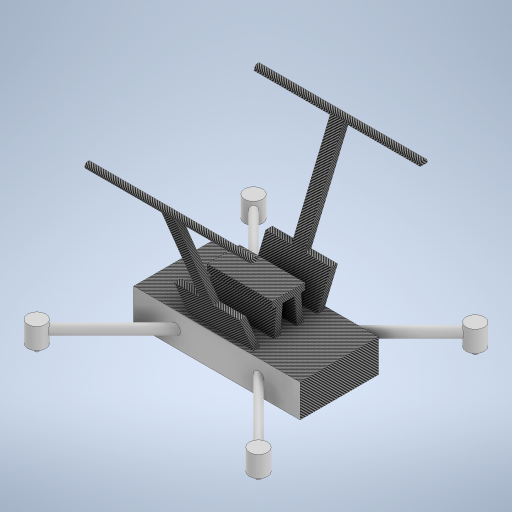
# Autodesk Inventor part: Drone_Model
Saved by Autodesk Inventor 2023 (Build 270158000, 158)
## iProperties
Created: 2022-11-14
Part Number: Drone_Model
Material: Generic
Document SubType Name: Modeling
Designer: cheng
Density: 1 g/cm^3
Appearance: Default
Mass: 1853.08 g
Surface Area: 1828.35 cm^2
Volume: 1853.08 cm^3
Author: cheng
Autodesk Inventor part; units mm, degrees
ref_plane "YZ Plane" through (0, 0, 0) normal (1, 0, 0) x (0, 1, 0)
ref_plane "XZ Plane" through (0, 0, 0) normal (0, 1, 0) x (-1, 0, 0)
sketch "Sketch4" plane through (0, 0, 0) normal (0, 1, 0) x (-1, 0, 0)
  line L0 (-102.6818, 131.0909) -> (-102.6818, 58.0909) construction
  line L1 (24.8182, 125) -> (-230.1818, 125)
  line L2 (-230.1818, 125) -> (-230.1818, 135)
  line L3 (-230.1818, 135) -> (24.8182, 135)
  line L4 (24.8182, 135) -> (24.8182, 125)
  line L5 (24.8182, 125) -> (-230.1818, 135) construction
  line L6 (-230.1818, 125) -> (24.8182, 135) construction
  line L7 (0, 0) -> (36.133, 0) construction
  line L8 (24.8182, -125) -> (-230.1818, -125)
  line L9 (-230.1818, -125) -> (-230.1818, -135)
  line L10 (-230.1818, -135) -> (24.8182, -135)
  line L11 (24.8182, -135) -> (24.8182, -125)
  line L12 (24.8182, -125) -> (-230.1818, -135) construction
  line L13 (-230.1818, -125) -> (24.8182, -135) construction
  point P0 (-102.6818, 130)
  dimension "d4" = 10
  dimension "d6" = 250
  dimension "d7" = 255
  constraints: 28 end point, 4 symmetric about line, 2 horizontal, 2 midpoint, 2 parallel, 1 perpendicular, 1 point on line, 1 vertical
  measures "d4" distance of L3.end L1.start
  measures "d6" distance between parallel lines of L8 L1
  measures "d7" distance of L2.end L3.end
extrude "Extrusion2" add sketch "Sketch4" along normal blind 10
sketch "Sketch9" plane through (230.1818, 0, -125) normal (1, 0, 0) x (0, 0, -1)
  line L0 (-125, 0) -> (-125, -106.9842) construction
  line L1 (10, 0) -> (10, 10) construction
  line L2 (0, 10) -> (10, 10) construction
  line L3 (10, 0) -> (0, 10) construction
  line L4 (0, 10) -> (10, 10) construction
  line L5 (10, 10) -> (0, 0) construction
  circle A0 centre (5, 5) radius 5
  line L6 (-260, 0) -> (-260, 10) construction
  line L7 (-250, 10) -> (-260, 10) construction
  line L8 (-260, 0) -> (-250, 10) construction
  line L9 (-250, 10) -> (-260, 10) construction
  line L10 (-260, 10) -> (-250, 0) construction
  circle A1 centre (-255, 5) radius 5
  constraints: 18 end point, 5 symmetric about line, 2 centre point, 1 collinear, 1 midpoint, 1 tangent, 1 vertical, 1 other
extrude "Extrusion3" cut sketch "Sketch9" against normal through all keep common part
sketch "Sketch10" plane through (230.1818, 5, -130) normal (1, 0, 0) x (0, 0, -1)
  circle A0 centre (0, 0) radius 5 construction
  line L0 (0, 5) -> (-260, 5)
  line L1 (-130, -5) -> (-130, 5) construction
  line L2 (-155, -155.4301) -> (-105, -155.4301)
  line L3 (-105, -155.4301) -> (-105, -145)
  line L4 (-105, -145) -> (-155, -145)
  line L5 (-155, -145) -> (-155, -155.4301)
  line L6 (-155, -155.4301) -> (-105, -145) construction
  line L7 (-105, -155.4301) -> (-155, -145) construction
  line L8 (-130, -150.215) -> (-130, -124.8826) construction
  dimension "d13" = 150
  dimension "d34" = 50
  constraints: 18 end point, 3 horizontal, 3 midpoint, 2 parallel, 1 collinear, 1 perpendicular, 1 vertical, 1 vertical alignment, 1 other
  measures "d13" distance between parallel lines of L4 L0
  measures "d34" distance of L2.start L2.end
extrude "Extrusion4" add sketch "Sketch10" against normal blind 255
sketch "Sketch11" plane through (230.1818, 5, -130) normal (1, 0, 0) x (0, 0, -1)
  circle A0 centre (0, 0) radius 5 projected
  line L0 (-155, -145) -> (-105, -145) projected
  line L1 (-130, 0) -> (-130, -145) construction
  line L2 (-130, -145) -> (-286.0792, -145) construction
  line L3 (-130, -145) -> (0, -145) construction
  circle A1 centre (-60, -145) radius 5
  circle A2 centre (-200, -145) radius 5
  line L4 (-55, -145) -> (4.6154, -1.9231)
  circle A3 centre (-260, 0) radius 5 projected
  line L5 (-190, -245.9934) -> (-70, -245.9934)
  line L6 (-70, -245.9934) -> (-70, -195.9934)
  line L7 (-70, -195.9934) -> (-190, -195.9934)
  line L8 (-190, -195.9934) -> (-190, -245.9934)
  line L9 (-190, -245.9934) -> (-70, -195.9934) construction
  line L10 (-70, -245.9934) -> (-190, -195.9934) construction
  line L11 (-130, -220.9934) -> (-130, -179.9046) construction
  line L12 (-55, -145) -> (-76.2472, -195.9934)
  line L13 (-5, 0) -> (-65, -145)
  line L14 (-65, -145) -> (-86.1007, -195.9934)
  line L15 (-255, 0) -> (-195, -145)
  line L16 (-263.5381, -3.533) -> (-205, -145)
  line L17 (-195, -145) -> (-173.8993, -195.9934)
  line L18 (-205, -145) -> (-183.8993, -195.9934)
  point P0 (-130, -5)
  dimension "d18" = 10
  dimension "d20" = 140
  dimension "d21" = 120
  dimension "d22" = 50
  constraints: 36 end point, 9 point on circle, 9 point on line, 5 collinear, 4 midpoint, 3 parallel, 2 centre point, 2 horizontal, 1 perpendicular, 1 symmetric about line, 1 vertical, 1 other
  measures "d18" diameter of A1
  measures "d20" distance of A2.centre A1.centre
  measures "d21" distance of L6.end L7.end
  measures "d22" distance of L7.end L5.start
extrude "Extrusion5" add sketch "Sketch11" against normal blind 255 contours A0 L4 A1 L13 | A1 L12 L13 | A1 L12 L7 L14 | L7 L6 L5 L8 | L7 L18 A2 L17 | A2 L18 L15 | A2 L16 A3 L15
sketch "Sketch12" plane through (-24.8182, 5, -130) normal (-1, 0, 0) x (0, 0, 1)
  line L0 (173.8993, -195.9934) -> (86.1007, -195.9934) projected
  line L1 (105, -155.4301) -> (155, -155.4301) projected
  line L2 (86.1007, -195.9934) -> (173.8993, -195.9934) projected
  line L3 (152.374, -195.9934) -> (149.1071, -155.4301)
  line L4 (142.3416, -195.9934) -> (139.0748, -155.4301)
  line L5 (155, -155.4301) -> (105, -155.4301) projected
  line L6 (255, 0) -> (173.8993, -195.9934) projected
  line L7 (86.1007, -195.9934) -> (5, 0) projected
  line L8 (173.8993, -195.9934) -> (105, -155.4301) construction
  line L9 (155, -155.4301) -> (86.1007, -195.9934) construction
  line L10 (130, -170.1484) -> (130, -155.4301) construction
  line L11 (107.626, -195.9934) -> (110.8929, -155.4301)
  line L12 (117.6584, -195.9934) -> (120.9252, -155.4301)
  point P0 (130, -5)
  point P1 (107.626, -195.9934)
  point P2 (117.6584, -195.9934)
  dimension "d25" = 10
  constraints: 14 end point, 6 point on line, 4 symmetric about line, 1 midpoint
  measures "d25" distance between parallel lines of L4 L3
extrude "Extrusion6" add sketch "Sketch12" against normal blind 255 contours L0 L4 L1 L3 | L0 L11 L1 L12
sketch "Sketch13" plane through (230.1818, -240.9934, -60) normal (0, 0, -1) x (-1, 0, 0)
  line L0 (0, 50) -> (255, 50) projected
  line L1 (0, 50) -> (0, 244.0703) projected
  line L2 (0, 50) -> (255, 50) projected
  line L3 (255, 244.0703) -> (255, 50) projected
  line L4 (0, 244.0703) -> (255, 244.0703) projected
  line L5 (0, 90.5633) -> (255, 90.5633) projected
  line L6 (0, 100.9934) -> (255, 100.9934) projected
  line L7 (0, 0) -> (255, 0) projected
  line L8 (0, 0) -> (0, 50) projected
  line L9 (255, 50) -> (255, 0) projected
  line L10 (255, 100.9934) -> (0, 244.0703) construction
  line L11 (1.2728, 100.9934) -> (255, 244.0703) construction
  line L12 (138.1364, 100.9934) -> (118.1364, 100.9934)
  line L13 (118.1364, 100.9934) -> (118.1364, 244.0703)
  line L14 (118.1364, 244.0703) -> (138.1364, 244.0703)
  line L15 (138.1364, 244.0703) -> (138.1364, 100.9934)
  line L16 (138.1364, 100.9934) -> (118.1364, 244.0703) construction
  line L17 (118.1364, 100.9934) -> (138.1364, 244.0703) construction
  point P0 (230.1818, 240.9934)
  point P1 (128.1364, 172.5318)
  point P2 (138.1364, 100.9934)
  point P3 (118.1364, 100.9934)
  dimension "d28" = 20
  constraints: 16 end point, 3 midpoint, 2 parallel, 2 point on line, 1 horizontal, 1 perpendicular
  measures "d28" distance of L13.end L14.end
extrude "Extrusion7" cut sketch "Sketch13" along normal mid plane 434.75 contours L1 L4 L13 L6 | L6 L15 L4 L3
sketch "Sketch14" plane through (230.1818, -240.9934, -60) normal (0, 0, -1) x (-1, 0, 0)
  line L0 (0, 50) -> (255, 50) projected
  line L1 (255, 100.9934) -> (255, 50) projected
  line L2 (255, 50) -> (255, 0) projected
  line L3 (255, 100.9934) -> (138.1364, 100.9934) projected
  line L4 (0, 0) -> (255, 0) projected
  line L5 (0, 0) -> (0, 50) projected
  line L6 (0, 90.5633) -> (255, 90.5633) projected
  line L7 (0, 100.9934) -> (118.1364, 100.9934) projected
  line L8 (0, 100.9934) -> (0, 50) projected
  line L9 (118.1364, 100.9934) -> (138.1364, 100.9934)
  line L10 (128.1364, 88.0174) -> (128.1364, 65.5782) construction
  line L11 (255, 90.5633) -> (0, 100.9934) construction
  line L12 (0, 90.5633) -> (255, 100.9934) construction
  line L13 (127.5, 95.7783) -> (127.5, 90.5633) construction
  line L14 (0, 50) -> (255, 50) projected
  line L15 (77.5, 50) -> (177.5, 50)
  line L16 (177.5, 50) -> (177.5, 100.9934)
  line L17 (177.5, 100.9934) -> (77.5, 100.9934)
  line L18 (77.5, 100.9934) -> (77.5, 50)
  line L19 (177.5, 50) -> (77.5, 100.9934) construction
  line L20 (177.5, 100.9934) -> (77.5, 50) construction
  line L21 (127.5, 75.4967) -> (127.5, 84.9841) construction
  point P0 (230.1818, 240.9934)
  point P1 (77.5, 50)
  point P2 (77.5, 100.9934)
  point P3 (177.5, 100.9934)
  dimension "d31" = 100
  constraints: 24 end point, 3 midpoint, 2 collinear, 2 horizontal, 2 parallel, 2 perpendicular, 2 vertical, 1 point on line
  measures "d31" distance between parallel lines of L18 L16
extrude "Extrusion8" cut sketch "Sketch14" along normal mid plane 434.75 contours L8 L6 L18 L0 | L8 L7 L18 L6 | L16 L6 L1 L0 | L16 L3 L1 L6
sketch "Sketch15" plane through (230.1818, -240.9934, -60) normal (0, 0, -1) x (-1, 0, 0)
  line L0 (0, 0) -> (0, 50) projected
  line L1 (0, 0) -> (255, 0) projected
  line L2 (255, 50) -> (255, 0) projected
  line L3 (0, 50) -> (255, 50) projected
  line L4 (0, 25) -> (255, 25) construction
  line L5 (77.5, 50) -> (177.5, 50) construction
  line L6 (127.5, 50) -> (127.5, 0) construction
  line L7 (127.5, 25) -> (0, 25) construction
  line L8 (127.5, 25) -> (255, 25) construction
  line L9 (63.75, 25) -> (63.75, 50) construction
  line L10 (63.75, 25) -> (63.75, 0) construction
  line L11 (191.25, 25) -> (191.25, 50) construction
  line L12 (191.25, 25) -> (191.25, 0) construction
  circle A0 centre (63.75, 25) radius 8
  circle A1 centre (191.25, 25) radius 8
  point P0 (230.1818, 240.9934)
  dimension "d35" = 16
  dimension "d36" = 16
  constraints: 16 end point, 7 midpoint, 6 point on line, 4 coincident, 2 centre point, 2 collinear, 2 perpendicular
  measures "d35" diameter of A0
  measures "d36" diameter of A1
sketch "Sketch17" plane through (230.1818, -240.9934, 60) normal (0, 0, 1) x (1, 0, 0)
  line L0 (0, 50) -> (0, 0) projected
  line L1 (0, 50) -> (-255, 50) projected
  line L2 (-255, 0) -> (-255, 50) projected
  line L3 (0, 0) -> (-255, 0) projected
  circle A0 centre (-63.75, 25) radius 8 projected
  circle A1 centre (-191.25, 25) radius 8 projected
  line L4 (0, 25) -> (-255, 25) construction
  line L5 (-191.25, 25) -> (-191.25, 50) construction
  line L6 (-191.25, 25) -> (-191.25, 0) construction
  line L7 (-127.5, 50) -> (-127.5, 0) construction
  line L8 (-63.75, 25) -> (-63.75, 0) construction
  line L9 (-63.75, 25) -> (-63.75, 50) construction
  point P0 (-230.1818, 240.9934)
ref_plane "Work Plane1" through (230.1818, -215.9934, -60) normal (0, -1, 0) x (-1, 0, 0)
sketch "Sketch18" plane through (230.1818, -215.9934, -60) normal (0, -1, 0) x (-1, 0, 0)
  line L0 (71.75, 0) -> (55.75, 0) projected
  line L1 (199.25, 0) -> (183.25, 0) projected
  line L2 (191.25, 0) -> (297.316, 106.066)
  line L3 (63.75, 0) -> (-42.316, 106.066)
  line L4 (183.25, -120) -> (199.25, -120) projected
  line L5 (55.75, -120) -> (71.75, -120) projected
  line L6 (191.25, -120) -> (297.316, -226.066)
  line L7 (63.75, -120) -> (-42.316, -226.066)
  point P0 (230.1818, -60)
  dimension "d47" = 150
  dimension "d49" = 45
  dimension "d50" = 45
  dimension "d51" = 45
  dimension "d52" = 45
  dimension "d53" = 150
  dimension "d54" = 150
  dimension "d55" = 150
  constraints: 8 end point, 4 midpoint
  measures "d47" distance of L7.start L7.end
  measures "d49" angle of L4 L6
  measures "d50" angle of L5 L7
  measures "d51" angle of L0 L3
  measures "d52" angle of L1 L2
  measures "d53" distance of L2.start L2.end
  measures "d54" distance of L3.start L3.end
  measures "d55" distance of L6.start L6.end
sweep "Sweep1" add profiles "Sketch17" path "Sketch18" path curves L6 contours A1
sweep "Sweep2" add profiles "Sketch17" path "Sketch18" path curves L7 contours A0
sweep "Sweep3" add profiles "Sketch15" path "Sketch18" path curves L2 contours A1
sweep "Sweep4" add profiles "Sketch15" path "Sketch18" path curves L3 contours A0
sketch "Sketch19" plane through (230.1818, -215.9934, -60) normal (0, -1, 0) x (-1, 0, 0)
  line L0 (-50.316, -226.066) -> (-34.316, -226.066) projected
  line L1 (-34.316, 106.066) -> (-50.316, 106.066) projected
  line L2 (305.316, 106.066) -> (289.316, 106.066) projected
  line L3 (289.316, -226.066) -> (305.316, -226.066) projected
  circle A0 centre (297.316, -226.066) radius 13.85
  circle A1 centre (297.316, 106.066) radius 13.85
  circle A2 centre (-42.316, 106.066) radius 13.85
  circle A3 centre (-42.316, -226.066) radius 13.85
  point P0 (230.1818, -60)
  dimension "d64" = 27.7
  dimension "d65" = 27.7
  dimension "d66" = 27.7
  dimension "d67" = 27.7
  constraints: 4 centre point, 4 midpoint
  measures "d64" diameter of A3
  measures "d65" diameter of A2
  measures "d66" diameter of A1
  measures "d67" diameter of A0
extrude "Extrusion9" add sketch "Sketch19" along normal blind 19 and the other way blind 13
sketch "Sketch20" plane through (272.4978, -234.9934, 166.066) normal (0, -1, 0) x (1, 0, 0)
  circle A0 centre (0, 0) radius 13.85 projected
  circle A1 centre (0, -332.132) radius 13.85 projected
  circle A2 centre (-339.632, -332.132) radius 13.85 projected
  circle A3 centre (-339.632, 0) radius 13.85 projected
  circle A4 centre (0, 0) radius 3
  circle A5 centre (0, -332.132) radius 3
  circle A6 centre (-339.632, -332.132) radius 3
  circle A7 centre (-339.632, 0) radius 3
  point P0 (-272.4978, -166.066)
  dimension "d72" = 6
  dimension "d73" = 6
  dimension "d74" = 6
  dimension "d75" = 6
  constraints: 4 centre point, 4 coincident
  measures "d72" diameter of A4
  measures "d73" diameter of A7
  measures "d74" diameter of A6
  measures "d75" diameter of A5
extrude "Extrusion10" add sketch "Sketch20" along normal blind 9.5 contours A4 | A5 | A6 | A7
sketch "Sketch21" plane through (272.4978, -234.9934, 166.066) normal (0, -1, 0) x (1, 0, 0)
  circle A0 centre (0, 0) radius 3 projected
  circle A1 centre (0, -332.132) radius 3 projected
  circle A2 centre (-339.632, 0) radius 3 projected
  circle A3 centre (-339.632, -332.132) radius 3 projected
  circle A4 centre (0, 0) radius 4.5
  circle A5 centre (0, -332.132) radius 3 projected
  circle A6 centre (0, -332.132) radius 4.5
  circle A7 centre (-339.632, -332.132) radius 3 projected
  circle A8 centre (-339.632, -332.132) radius 4.5
  circle A9 centre (-339.632, 0) radius 3 projected
  circle A10 centre (-339.632, 0) radius 4.5
  point P0 (-272.4978, -166.066)
  dimension "d78" = 9
  dimension "d79" = 9
  dimension "d80" = 9
  dimension "d81" = 9
  constraints: 4 centre point, 4 coincident
  measures "d78" diameter of A4
  measures "d79" diameter of A10
  measures "d80" diameter of A8
  measures "d81" diameter of A6
extrude "Extrusion11" add sketch "Sketch21" along normal blind 4 contours A0 | A1 | A2 | A3 | A4 | A6 | A8 | A10
equation "\"d53\" = d47"
equation "\"d54\" = d47"
equation "\"d55\" = d47"
equation "\"d65\" = d64"
equation "\"d66\" = d64"
equation "\"d67\" = d64"
equation "\"d73\" = d72"
equation "\"d74\" = d72"
equation "\"d75\" = d72"
equation "\"d79\" = d78"
equation "\"d80\" = d78"
equation "\"d81\" = d78"
body "Solid2"
